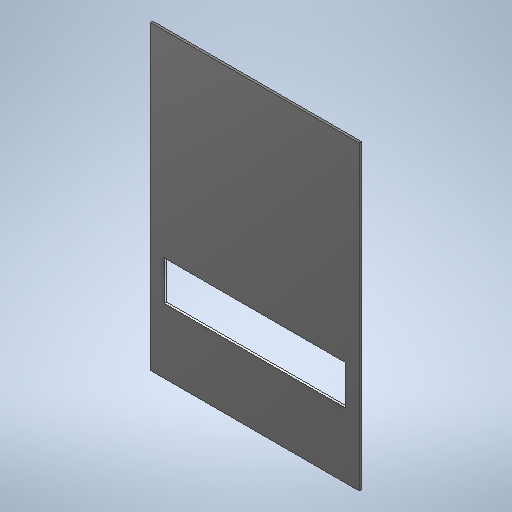
# Autodesk Inventor part: Foam Sheet Front
Saved by Autodesk Inventor 2026.2 (Build 302298010, 298A)
## iProperties
Created: 2026-06-07
Part Number: Foam Sheet Front
Material: PVC-Piping
Document SubType Name: Modeling
Designer: chanh
Density: 1.4 g/cm^3
Appearance: Smooth - White
Author: chanh
Autodesk Inventor part; units mm, degrees
ref_plane "YZ Plane" through (0, 0, 0) normal (1, 0, 0) x (0, 1, 0)
ref_plane "XZ Plane" through (0, 0, 0) normal (0, 1, 0) x (-1, 0, 0)
ref_plane "XY Plane" through (0, 0, 0) normal (0, 0, 1) x (1, 0, 0)
sketch "Sketch1" plane through (0, 0, 0) normal (0, 0, 1) x (1, 0, 0)
  line L0 (-225, -325) -> (225, -325)
  line L1 (225, -325) -> (225, 325)
  line L2 (225, 325) -> (-225, 325)
  line L3 (-225, 325) -> (-225, -325)
  line L4 (-225, -325) -> (225, 325) construction
  line L5 (225, -325) -> (-225, 325) construction
  line L6 (-195, -185) -> (195, -185)
  line L7 (195, -185) -> (195, -100)
  line L8 (195, -100) -> (-195, -100)
  line L9 (-195, -100) -> (-195, -185)
  line L10 (-195, -185) -> (195, -100) construction
  line L11 (195, -185) -> (-195, -100) construction
  point P0 (0, 0)
  point P1 (0, -142.5)
  dimension "d0" = 450
  dimension "d1" = 650
  dimension "d4" = 140
  dimension "d5" = 225
  dimension "d6" = 390
  constraints: 24 end point, 4 midpoint, 4 parallel, 2 horizontal, 2 perpendicular, 1 vertical alignment
  measures "d0" distance of L1.end L2.end
  measures "d1" distance of L0.end L1.end
  measures "d4" distance between parallel lines of L0 L6
  measures "d5" distance between parallel lines of L8 L0
  measures "d6" distance of L7.end L8.end
extrude "Extrusion1" add sketch "Sketch1" along normal blind 5
body "Solid1"
